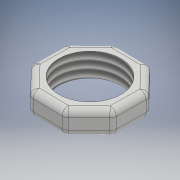
# Autodesk Inventor part: AnnishBT
Saved by Autodesk Inventor 2017 (Build 210142000, 142)
## iProperties
Created: 2018-02-22
Part Number: AnnishBT
Material: Generic
Document SubType Name: Modeling
Designer: CMRU-CAD-PC 7
Density: 1 g/cm^3
Appearance: Default
Author: CMRU-CAD-PC 7
Autodesk Inventor part; units mm, degrees
ref_plane "YZ Plane" through (0, 0, 0) normal (1, 0, 0) x (0, 1, 0)
ref_plane "XZ Plane" through (0, 0, 0) normal (0, 1, 0) x (-1, 0, 0)
ref_plane "XY Plane" through (0, 0, 0) normal (0, 0, 1) x (1, 0, 0)
sketch "Sketch1" plane through (0, 0, 0) normal (0, 0, 1) x (1, 0, 0)
  circle A0 centre (0, 0) radius 8
  line L0 (10.6699, -4.6008) -> (4.2915, -10.798)
  line L1 (4.2915, -10.798) -> (-4.6008, -10.6699)
  line L2 (-4.6008, -10.6699) -> (-10.798, -4.2915)
  line L3 (-10.798, -4.2915) -> (-10.6699, 4.6008)
  line L4 (-10.6699, 4.6008) -> (-4.2915, 10.798)
  line L5 (-4.2915, 10.798) -> (4.6008, 10.6699)
  line L6 (4.6008, 10.6699) -> (10.798, 4.2915)
  line L7 (10.798, 4.2915) -> (10.6699, -4.6008)
  dimension "d0" = 16
  constraints: 16 end point, 2 coincident, 1 centre point, 17 other
  measures "d0" diameter of A0
extrude "Extrusion1" add sketch "Sketch1" along normal blind 6
fillet "Fillet1" radius 1.6 23 edges at (7.4807, -7.6994, 6) (10.6699, -4.6008, 3) (10.7339, -0.1546, 6) (10.798, 4.2915, 3) (4.2915, -10.798, 3) (-0.1546, -10.7339, 6) (-4.6008, -10.6699, 3) (-0.1546, -10.7339, 0) (10.7339, -0.1546, 0) (7.4807, -7.6994, 0) (7.6994, 7.4807, 0) (0.1546, 10.7339, 0) (-7.4807, 7.6994, 0) (-10.7339, 0.1546, 0) (-7.6994, -7.4807, 0) (-4.2915, 10.798, 3) (-10.6699, 4.6008, 3) (-10.798, -4.2915, 3) (7.6994, 7.4807, 6) (0.1546, 10.7339, 6) (-7.6994, -7.4807, 6) (-10.7339, 0.1546, 6) (-7.4807, 7.6994, 6)
thread "Thread1" size "M16x2" class "6H" standard "ISO Metric profile" full length
body "Solid1"
